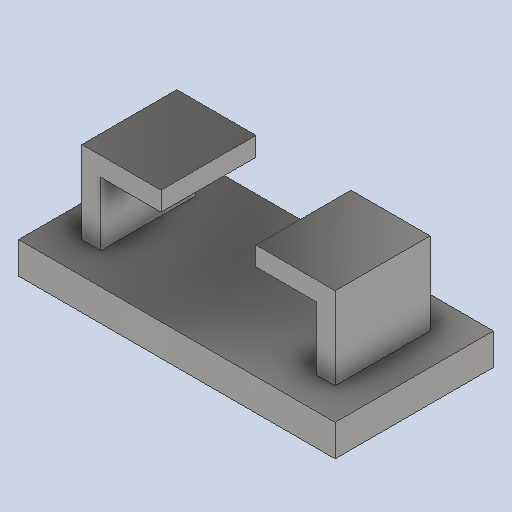
# Autodesk Inventor part: holder sensor
Saved by Autodesk Inventor 2025 (Build 290162000, 162)
## iProperties
Created: 2024-10-01
Part Number: holder sensor
Material: Generic
Document SubType Name: Modeling
Designer: DMIADX
Density: 1 g/cm^3
Appearance: Steel - Polished
Author: DMIADX
Autodesk Inventor part; units mm, degrees
ref_plane "YZ Plane" through (0, 0, 0) normal (1, 0, 0) x (0, 1, 0)
ref_plane "XZ Plane" through (0, 0, 0) normal (0, 1, 0) x (-1, 0, 0)
ref_plane "XY Plane" through (0, 0, 0) normal (0, 0, 1) x (1, 0, 0)
sketch "Sketch1" plane through (0, 0, 0) normal (0, 1, 0) x (-1, 0, 0)
  line L0 (-50, -25) -> (50, -25)
  line L1 (50, -25) -> (50, 25)
  line L2 (50, 25) -> (-50, 25)
  line L3 (-50, 25) -> (-50, -25)
  line L4 (-50, -25) -> (50, 25) construction
  line L5 (50, -25) -> (-50, 25) construction
  point P0 (0, 0)
  dimension "d0" = 100
  dimension "d1" = 50
  constraints: 12 end point, 2 midpoint, 2 parallel, 1 horizontal, 1 perpendicular
  measures "d0" distance of L2.end L1.end
  measures "d1" distance of L1.end L0.end
extrude "Extrusion1" add sketch "Sketch1" along normal blind 10
sketch "Sketch2" plane through (0, 0, 0) normal (0, 0, 1) x (1, 0, 0)
  line L0 (-50, 10) -> (50, 10) projected
  line L1 (31.5957, 10) -> (-31.5209, 10)
  line L2 (15, 10) -> (-15, 10)
  line L3 (-15, 10) -> (-15, 36)
  line L4 (-15, 36) -> (15, 36)
  line L5 (15, 36) -> (15, 10)
  line L6 (15, 10) -> (-15, 36) construction
  line L7 (-15, 10) -> (15, 36) construction
  line L8 (34, 30) -> (-34, 30)
  line L9 (-34, 30) -> (-34, 10)
  line L10 (-34, 10) -> (34, 10)
  line L11 (34, 10) -> (34, 30)
  line L12 (34, 30) -> (-34, 10) construction
  line L13 (-34, 30) -> (34, 10) construction
  line L14 (40, 36) -> (-40, 36)
  line L15 (-40, 36) -> (-40, 10)
  line L16 (-40, 10) -> (40, 10)
  line L17 (40, 10) -> (40, 36)
  line L18 (40, 36) -> (-40, 10) construction
  line L19 (-40, 36) -> (40, 10) construction
  line L20 (-50, 0) -> (50, 0) projected
  point P0 (0, 0)
  point P1 (0, 23)
  point P2 (0, 20)
  point P3 (0, 23)
  point P4 (-34, 20)
  point P5 (0, 0)
  point P6 (0, 0)
  point P7 (0, 0)
  point P8 (0, 10)
  point P9 (40, 10)
  point P10 (15, 36)
  point P11 (15, 30)
  point P12 (34, 10)
  point P13 (-34, 10)
  point P14 (-15, 30)
  point P15 (-15, 36)
  dimension "d5" = 80
  dimension "d7" = 0
  dimension "d8" = 6
  dimension "d9" = 30
  dimension "d10" = 20
  dimension "d13" = 68
  constraints: 38 end point, 12 midpoint, 6 parallel, 4 horizontal, 3 perpendicular, 3 point on line, 3 vertical alignment
  measures "d5" distance between parallel lines of L17 L15
  measures "d7" distance between parallel lines of L14 L4
  measures "d8" distance between parallel lines of L14 L8
  measures "d9" distance between parallel lines of L5 L3
  measures "d10" distance between parallel lines of L10 L8
  measures "d13" distance of L8.start L8.end
extrude "Extrusion2" add sketch "Sketch2" along normal mid plane 30 contours L15 L14 L3 L8 L9 L0 | L14 L17 L0 L11 L8 L5
body "Solid1"
